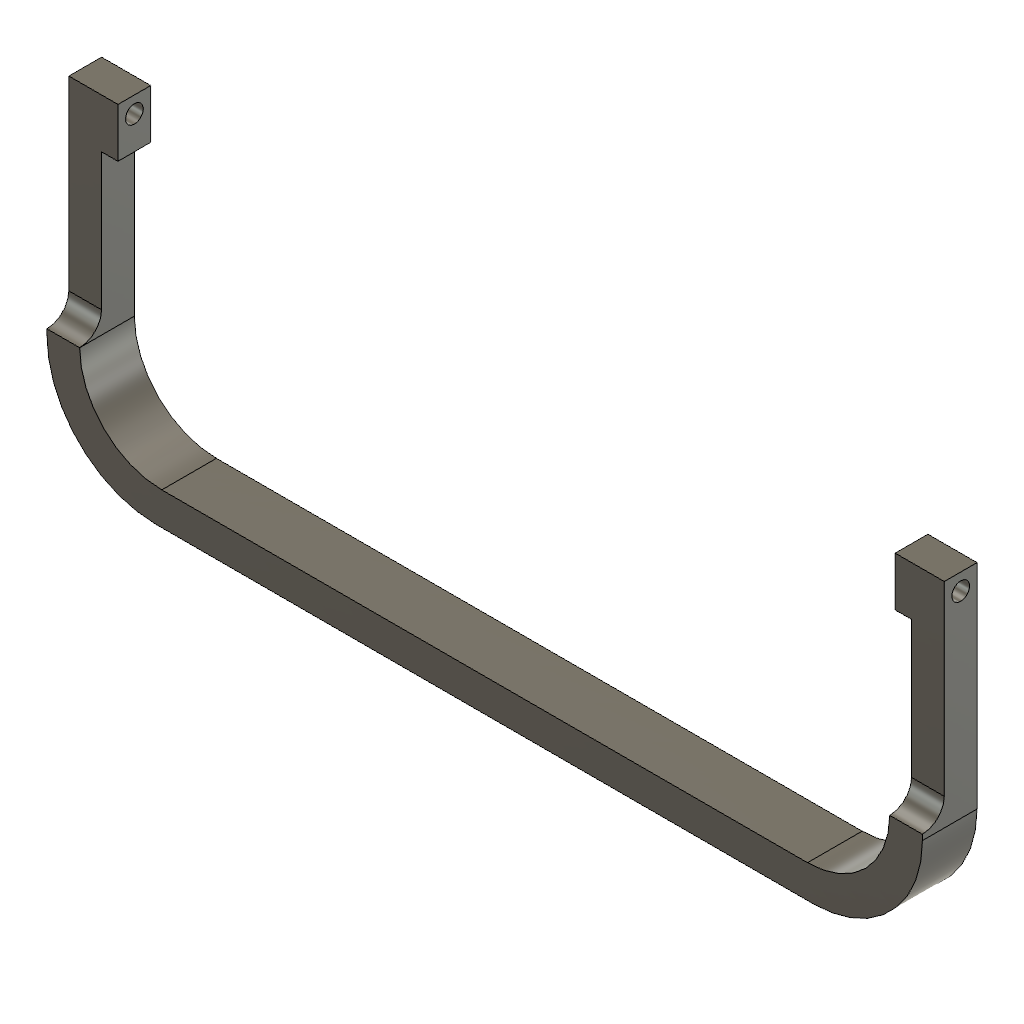
TankBot Bumper for Switch (Autodesk Fusion 360 design; units mm, degrees)
Autodesk Fusion 360 part; units mm, degrees
box "BoxPrimitive1" add length 10 width 160 height 3 placed x (0, 0, 1) y (1, 0, 0) z (0, 1, 0) at (0, 0, 0)
box "BoxPrimitive2" add length 10 width 9 height 56 placed x (0, 0, 1) y (1, 0, 0) z (0, 1, 0) at (151, 3, 0)
box "BoxPrimitive3" add length 10 width 9 height 56 placed x (0, 0, 1) y (1, 0, 0) z (0, 1, 0) at (0, 3, 0)
extrude "Extrude1" add 1 faces at (103.6667, 3, 3.3333) along direction (0, 1, 0) blind 3
extrude "Extrude2" cut 1 faces at (9, 23.6667, 3.3333) along direction (-1, 0, 0) blind 3
extrude "Extrude3" cut 1 faces at (151, 23.6667, 3.3333) along direction (1, 0, 0) blind 3
box "BoxPrimitive4" add length 9 width 10 height 3 placed x (0, -1, 0) y (0, 0, 1) z (-1, 0, 0) at (154, 59, 0)
box "BoxPrimitive5" add length 9 width 10 height 3 placed x (0, -1, 0) y (0, 0, -1) z (1, 0, 0) at (6, 59, 10)
hole "Hole1" at (160, 56, 3) direction (-1, 0, 0) diameter 3.25 depth 160 tip angle 180
box "BoxPrimitive6" cut length 29 width 6 height -4 placed x (0, 1, 0) y (-1, 0, 0) z (0, 0, 1) at (160, 21, 10)
fillet "Fillet1" radius 15 1 edges at (154, 6, 5)
fillet "Fillet2" radius 20 1 edges at (160, 0, 5)
extrude "Extrude5" cut 1 faces at (157, 56, 10) along direction (0, 0, -1) blind 4
box "BoxPrimitive7" cut length 29 width 6 height -4 placed x (0, -1, 0) y (1, 0, 0) z (0, 0, 1) at (0, 50, 10)
fillet "Fillet3" radius 20 1 edges at (0, 0, 5)
fillet "Fillet4" radius 15 1 edges at (6, 6, 5)
extrude "Extrude6" cut 1 faces at (3, 56, 10) along direction (0, 0, -1) blind 4
fillet "Fillet5" radius 4 1 edges at (3, 21, 6)
fillet "Fillet6" radius 4 1 edges at (157, 21, 6)
